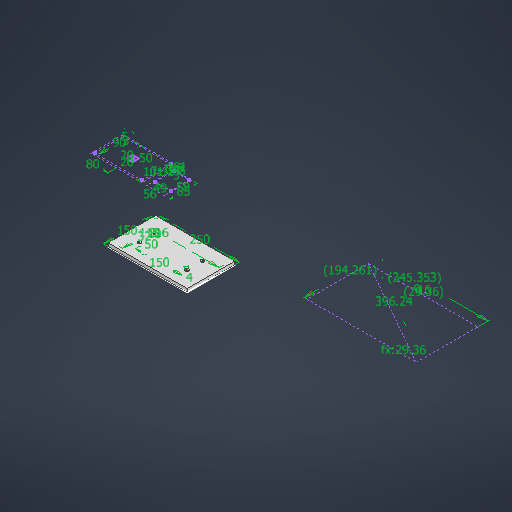
# Autodesk Inventor part: Main Mount
Saved by Autodesk Inventor 2025.1 (Build 291241000, 241)
## iProperties
Created: 2025-02-09
Part Number: Main Mount
Material: Generic
Document SubType Name: Modeling
Designer: jerem
Density: 1 g/cm^3
Appearance: Default
Author: jerem
Autodesk Inventor part; units mm, degrees
ref_plane "YZ Plane" through (0, 0, 0) normal (1, 0, 0) x (0, 1, 0)
ref_plane "XZ Plane" through (0, 0, 0) normal (0, 1, 0) x (-1, 0, 0)
ref_plane "XY Plane" through (0, 0, 0) normal (0, 0, 1) x (1, 0, 0)
sketch "Sketch1" plane through (0, 0, 0) normal (0, 1, 0) x (-1, 0, 0)
  line L0 (-74, 25) -> (76, 25) construction
  line L1 (76, 25) -> (76, -25) construction
  circle A0 centre (-74, 25) radius 2
  circle A1 centre (76, 25) radius 2
  circle A2 centre (76, -25) radius 2
  line L2 (-74, 25) -> (-74, -25) construction
  circle A3 centre (-74, -25) radius 2
  line L3 (108, 57.5) -> (-108, 57.5) construction
  line L4 (-108, 57.5) -> (-108, -57.5) construction
  line L5 (-108, -57.5) -> (108, -57.5) construction
  line L6 (108, -57.5) -> (108, 57.5) construction
  line L7 (108, 0) -> (76, 0) construction
  line L8 (-333.2556, -289.2611) -> (-678.6087, -289.2611) construction
  line L9 (-678.6087, -289.2611) -> (-678.6087, -95) construction
  line L10 (-678.6087, -95) -> (-333.2556, -95) construction
  line L11 (-333.2556, -95) -> (-333.2556, -289.2611) construction
  line L12 (-333.2556, -289.2611) -> (-678.6087, -95) construction
  line L13 (-488.8826, -290.1866) -> (-488.8826, -299.1866) construction
  line L14 (-488.8826, -299.1866) -> (-504.8826, -299.1866) construction
  line L15 (-488.8826, -290.1866) -> (-504.8826, -299.1866) construction
  line L16 (337.0989, -214.3276) -> (337.0989, -194.3276)
  line L17 (402.0989, -159.3276) -> (402.0989, -249.3276) construction
  circle A4 centre (402.0989, -159.3276) radius 1.5
  line L18 (407.0989, -254.3276) -> (407.0989, -153.3276) construction
  line L19 (402.0989, -249.3276) -> (252.0989, -249.3276) construction
  line L20 (246.0989, -254.3276) -> (407.0989, -254.3276) construction
  line L21 (407.0989, -153.3276) -> (246.0989, -153.3276) construction
  line L22 (252.0989, -159.3276) -> (402.0989, -159.3276) construction
  line L23 (317.0989, -214.3276) -> (337.0989, -214.3276)
  line L24 (317.0989, -194.3276) -> (317.0989, -214.3276)
  line L25 (317.0989, -214.3276) -> (337.0989, -194.3276) construction
  line L26 (337.0989, -214.3276) -> (317.0989, -194.3276) construction
  line L27 (337.0989, -194.3276) -> (317.0989, -194.3276)
  line L28 (246.0989, -153.3276) -> (246.0989, -254.3276) construction
  line L29 (252.0989, -249.3276) -> (252.0989, -159.3276) construction
  circle A5 centre (252.0989, -159.3276) radius 1.5
  circle A6 centre (252.0989, -249.3276) radius 1.5
  circle A7 centre (402.0989, -249.3276) radius 1.5
  line L30 (402.0989, -249.3276) -> (402.0989, -254.3276) construction
  line L31 (402.0989, -249.3276) -> (407.0989, -249.3276) construction
  line L32 (231.0989, -238.3276) -> (175.0989, -238.3276) construction
  line L33 (175.0989, -238.3276) -> (175.0989, -153.3276) construction
  line L34 (175.0989, -153.3276) -> (231.0989, -153.3276) construction
  line L35 (231.0989, -153.3276) -> (231.0989, -238.3276) construction
  line L36 (227.5989, -234.8276) -> (178.5989, -234.8276) construction
  line L37 (178.5989, -234.8276) -> (178.5989, -176.8276) construction
  line L38 (178.5989, -176.8276) -> (227.5989, -176.8276) construction
  line L39 (227.5989, -176.8276) -> (227.5989, -234.8276) construction
  circle A8 centre (227.5989, -234.8276) radius 1.5
  circle A9 centre (178.5989, -234.8276) radius 1.5
  circle A10 centre (227.5989, -176.8276) radius 1.5
  circle A11 centre (178.5989, -176.8276) radius 1.5
  line L40 (203.0989, -234.8276) -> (203.0989, -238.3276) construction
  line L41 (-125, 75) -> (125, 75)
  line L42 (125, 75) -> (125, -75)
  line L43 (125, -75) -> (-125, -75)
  line L44 (-125, -75) -> (-125, 75)
  line L45 (-125, 75) -> (125, -75) construction
  line L46 (125, 75) -> (-125, -75) construction
  line L47 (0, -57.5) -> (0, -75)
  line L48 (108, 0) -> (125, 0) construction
  circle A12 centre (76, -25) radius 5
  circle A13 centre (76, 25) radius 5
  circle A14 centre (-74, 25) radius 5
  circle A15 centre (-74, -25) radius 5
  point P0 (0, 0)
  point P1 (327.0989, -204.3276)
  dimension "d0" = 150
  dimension "d1" = 50
  dimension "d2" = 4
  dimension "d3" = 32
  dimension "d4" = 216
  dimension "d5" = 115
  dimension "d34" = 396.24
  dimension "d37" = 345.3531
  dimension "d39" = 9
  dimension "d40" = 16
  dimension "d41" = 29.358
  dimension "d42" = 29.358
  dimension "d43" = 194.2611
  dimension "d46" = 161
  dimension "d47" = 101
  dimension "d48" = 3
  dimension "d49" = 150
  dimension "d50" = 90
  dimension "d51" = 5
  dimension "d52" = 20
  dimension "d53" = 20
  dimension "d54" = 50
  dimension "d55" = 80
  dimension "d56" = 56
  dimension "d57" = 85
  dimension "d58" = 49
  dimension "d59" = 58
  dimension "d60" = 3
  dimension "d61" = 3.5
  dimension "d62" = 15
  dimension "d64" = 250
  dimension "d65" = 150
  dimension "d66" = 10
  constraints: 98 end point, 16 centre point, 16 parallel, 15 coincident, 12 equal radius, 12 perpendicular, 11 midpoint, 10 horizontal, 4 vertical, 3 point on line, 2 equal length
  measures "d0" distance of L0.start L1.start
  measures "d1" distance of L1.start L1.end
  measures "d2" diameter of A0
  measures "d3" distance between parallel lines of L6 L1
  measures "d4" distance of L4.end L5.end
  measures "d5" distance of L5.end L3.start
  measures "d34" distance of L8.start L9.end
  measures "d37" distance of L8.start L8.end
  measures "d39" distance of L13.start L13.end
  measures "d40" distance of L13.end L14.end
  measures "d41" angle of L14 L15
  measures "d42" angle of L10 L12
  measures "d43" distance of L10.end L8.start
  measures "d46" distance of L20.end L20.start
  measures "d47" distance of L20.start L21.end
  measures "d48" diameter of A7
  measures "d49" distance of L19.start L19.end
  measures "d50" distance of L22.end L19.start
  measures "d51" distance of L19.start L30.end
  measures "d52" distance of L24.start L25.end
  measures "d53" distance of L25.end L23.end
  measures "d54" distance from line of L20 point (327.099, -204.328)
  measures "d55" distance from line of L18 point (327.099, -204.328)
  measures "d56" distance of L34.start L35.start
  measures "d57" distance of L32.end L34.start
  measures "d58" distance of L38.start L39.start
  measures "d59" distance of L36.end L38.start
  measures "d60" diameter of A8
  measures "d61" distance between parallel lines of L32 L36
  measures "d62" distance between parallel lines of L28 L35
  measures "d64" distance of L42.end L43.end
  measures "d65" distance of L41.end L42.end
  measures "d66" diameter of A12
extrude "Extrusion2" add sketch "Sketch1" along normal blind 10 contours L41 L42 L43 L44 | A12 | A13 | A14 | A15
extrude "Extrusion3" add sketch "Sketch1" along normal blind 2 from surface at 10 contours A12 | A13 | A14 | A15
body "Solid2"
